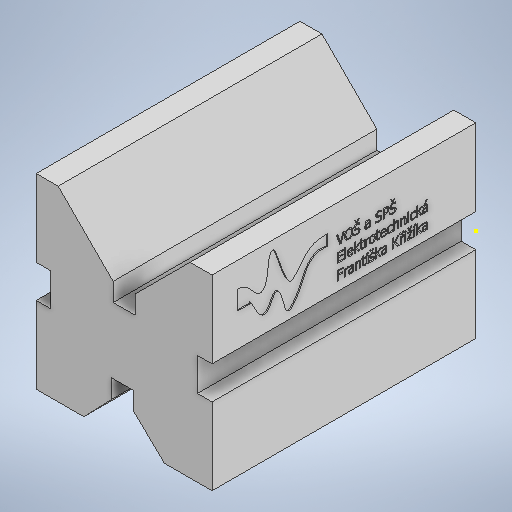
# Autodesk Inventor part: NECO
Saved by Autodesk Inventor 2025 (Build 290162000, 162)
## iProperties
Created: 2025-04-24
Part Number: NECO
Material: Všeobecné
Document SubType Name: Modeling
Designer: jakub
Density: 1 g/cm^3
Appearance: Výchozí
Author: jakub
Autodesk Inventor part; units mm, degrees
(part 1 of 2)
ref_plane "YZ Plane" through (0, 0, 0) normal (1, 0, 0) x (0, 1, 0)
ref_plane "XZ Plane" through (0, 0, 0) normal (0, 1, 0) x (-1, 0, 0)
ref_plane "XY Plane" through (0, 0, 0) normal (0, 0, 1) x (1, 0, 0)
sketch "Sketch1" plane through (0, 0, 0) normal (0, 0, 1) x (1, 0, 0)
  line L0 (0, 4.5) -> (0, 25.5)
  line L1 (0, 4.5) -> (4, 4.5)
  line L2 (4, 4.5) -> (4, 0)
  line L3 (0, 25.5) -> (6, 25.5)
  line L4 (0, 25.5) -> (6, 25.5)
  line L5 (26.7438, 0) -> (4, 0)
  line L6 (6, 25.5) -> (21, 10.5)
  line L7 (48, 4.5) -> (48, 25.5)
  line L8 (48, 4.5) -> (44, 4.5)
  line L9 (44, 4.5) -> (44, 0)
  line L10 (48, 25.5) -> (42, 25.5)
  line L11 (48, 25.5) -> (42, 25.5)
  line L12 (26.7438, 0) -> (44, 0)
  line L13 (42, 25.5) -> (27, 10.5)
  line L14 (24, 5.5) -> (21, 5.5)
  line L15 (21, 5.5) -> (21, 10.5)
  line L16 (24, 5.5) -> (27, 5.5)
  line L17 (27, 5.5) -> (27, 10.5)
  line L18 (4, 0) -> (4, -4.5)
  line L19 (4, -4.5) -> (0, -4.5)
  line L20 (0, 0) -> (0, -25.5)
  line L21 (0, -25.5) -> (48, -25.5)
  line L22 (44, 0) -> (44, -4.5)
  line L23 (44, -4.5) -> (48, -4.5)
  line L24 (48, -4.5) -> (48, -25.5)
  line L25 (0, -25.5) -> (13, -25.5)
  line L26 (13, -25.5) -> (35, -25.5)
  line L27 (20.5688, -12.5) -> (26.5688, -12.5)
  line L28 (13, -25.5) -> (20.5688, -17.6285)
  line L29 (26.5688, -17.3931) -> (35, -25.5)
  line L30 (23.5688, -12.5) -> (26.5688, -12.5)
  line L31 (26.5688, -12.5) -> (26.5688, -17.3931)
  line L32 (23.5688, -12.5) -> (20.5688, -12.5)
  line L33 (20.5688, -12.5) -> (20.5688, -17.6285)
  point P0 (23.7438, 7.7562)
  point P1 (24.2562, 7.7562)
  point P2 (24, -25.5)
  dimension "d0" = 25.5
  dimension "d1" = 4.5
  dimension "d3" = 6
  dimension "d10" = 90
  dimension "d14" = 4.5
  dimension "d15" = 25.5
  dimension "d16" = 48
  dimension "d17" = 13
  dimension "d18" = 22
  dimension "d22" = 90
  dimension "d25" = 6
  dimension "d26" = 13
  constraints: 68 end point, 9 perpendicular, 4 vertical, 3 midpoint, 3 point on line, 1 horizontal, 1 parallel
  measures "d0" distance of L20.start L0.end
  measures "d1" distance of L0.start L20.start
  measures "d3" distance of L3.end L0.end
  measures "d10" angle of L13 L6
  measures "d14" distance of L2.end L18.end
  measures "d15" distance of L20.start L20.end
  measures "d16" distance of L20.end L21.end
  measures "d17" distance of L20.end L25.end
  measures "d18" distance of L25.end L26.end
  measures "d22" angle of L28 L29
  measures "d25" distance of L16.end L14.end
  measures "d26" vertical distance of point (24, -25.5) point (23.569, -12.5)
extrude "Extrusion1" add sketch "Sketch1" along normal blind 72 contours L0 L3 L6 L15 L14 L16 L17 L13 L10 L7 L8 L9 L12 L5 L2 L1 | L5 L12 L22 L23 L24 L21 L29 L31 L27 L33 L28 L20 L19 L18
sketch "Sketch2" plane through (48, 4.5, 0) normal (1, 0, 0) x (0, 0, -1)
  point P0 (0, -4.5)
sketch "Sketch3" plane through (48, 4.5, 0) normal (1, 0, 0) x (0, 0, -1)
  point P0 (0, -4.5)
sketch "Sketch4" plane through (48, 4.5, 0) normal (1, 0, 0) x (0, 0, -1)
  line L0 (-113.7107, -9.1666) -> (-61.0617, -9.1666) construction
  line L1 (-61.0617, -9.1666) -> (-61.0617, -46.8985) construction
  line L2 (-61.0617, -46.8985) -> (-113.7107, -46.8985) construction
  line L3 (-113.7107, -46.8985) -> (-113.7107, -9.1666) construction
  line L4 (-65, 14) -> (-65, 9)
  line L5 (-65, 9) -> (-61.5478, 9)
  line L6 (-40, 12) -> (-42.9346, 12.1178)
  line L7 (-47.0264, 7.7112) -> (-45.9195, 10.8139) construction
  line L8 (-45.9195, 10.8139) -> (-44.0057, 11.8143) construction
  line L9 (-44.0057, 11.8143) -> (-42.9346, 12) construction
  line L10 (-42.9346, 12) -> (-42.9346, 12.1178) construction
  spline S0 degree 4 poles (-47.0264, 7.7112) (-45.9195, 10.8139) (-44.0057, 11.8143) (-42.9346, 12) (-42.9346, 12.1178) knots 1 1 1 1 1 2 2 2 2 2
  spline S1 degree 4 poles (-61.5478, 9) (-61.7679, 11.3374) (-57.3488, -3.3323) (-55.3925, 13.3367) (-52.3539, 5.2468) (-51.4968, -1.6929) (-46.4748, 8.2553) (-46.8368, 8.3647) (-46.4946, 9) knots 0 0 0 0 0 0.346923 0.494972 0.656933 0.800083 1 1 1 1 1
  line L11 (-42.9346, 12) -> (-40.3861, 12.0155)
  line L12 (-40.3861, 12.0155) -> (-40.3861, 15.0416)
  line L13 (-40.3861, 15.0416) -> (-41.6603, 15.0416) construction
  line L14 (-41.6603, 15.0416) -> (-43.7781, 14.867) construction
  line L15 (-43.7781, 14.867) -> (-44.6658, 14.328) construction
  line L16 (-44.6658, 14.328) -> (-46.302, 13.2956) construction
  line L17 (-46.302, 13.2956) -> (-48.14, 11.0974) construction
  line L18 (-48.14, 11.0974) -> (-49.7307, 9) construction
  line L19 (-49.7307, 9) -> (-50.3422, 8.6804) construction
  line L20 (-50.3422, 8.6804) -> (-50.9722, 8.9051) construction
  line L21 (-50.9722, 8.9051) -> (-52.1436, 10.724) construction
  line L22 (-52.1436, 10.724) -> (-53.3658, 14.2638) construction
  line L23 (-53.3658, 14.2638) -> (-54.7945, 18.2323) construction
  line L24 (-54.7945, 18.2323) -> (-55.2231, 18.645) construction
  line L25 (-55.2231, 18.645) -> (-55.6237, 18.645) construction
  line L26 (-55.6237, 18.645) -> (-56.0485, 18.2799) construction
  line L27 (-56.0485, 18.2799) -> (-56.5247, 17.2322) construction
  line L28 (-56.5247, 17.2322) -> (-56.7946, 13.8194) construction
  line L29 (-56.7946, 13.8194) -> (-57.2685, 11.365) construction
  line L30 (-57.2685, 11.365) -> (-58.1756, 10.2319) construction
  line L31 (-58.1756, 10.2319) -> (-58.8495, 10.1151) construction
  line L32 (-58.8495, 10.1151) -> (-59.4762, 10.1151) construction
  line L33 (-59.4762, 10.1151) -> (-60.4296, 11.1367) construction
  line L34 (-60.4296, 11.1367) -> (-61.8566, 12.8776) construction
  line L35 (-61.8566, 12.8776) -> (-63.0012, 13.74) construction
  line L36 (-63.0012, 13.74) -> (-64.3971, 14.238) construction
  line L37 (-64.3971, 14.238) -> (-65, 14.1232) construction
  spline S2 degree 4 poles (-40.3861, 15.0416) (-41.6603, 15.0416) (-43.7781, 14.867) (-44.6658, 14.328) (-46.302, 13.2956) (-48.14, 11.0974) (-49.7307, 9) (-50.3422, 8.6804) (-50.9722, 8.9051) (-52.1436, 10.724) (-53.3658, 14.2638) (-54.7945, 18.2323) (-55.2231, 18.645) (-55.6237, 18.645) (-56.0485, 18.2799) (-56.5247, 17.2322) (-56.7946, 13.8194) (-57.2685, 11.365) (-58.1756, 10.2319) (-58.8495, 10.1151) (-59.4762, 10.1151) (-60.4296, 11.1367) (-61.8566, 12.8776) (-63.0012, 13.74) (-64.3971, 14.238) (-65, 14.1232) knots 1 1 1 1 1 2 3 4 5 6 7 8 9 10 11 12 13 14 15 16 17 18 19 20 21 22 23 23 23 23 23
  line L38 (-65, 14.1232) -> (-65, 14)
  line L39 (-37.9985, 14.2982) -> (-1.01, 14.2982) construction
  line L40 (-1.01, 14.2982) -> (-1.01, 3.2238) construction
  line L41 (-1.01, 3.2238) -> (-37.9985, 3.2238) construction
  line L42 (-37.9985, 3.2238) -> (-37.9985, 14.2982) construction
  line L43 (-35.899, 13.3431) -> (-36.7738, 10.8031)
  line L44 (-36.7738, 10.8031) -> (-37.1381, 10.8031)
  line L45 (-37.1381, 10.8031) -> (-38.0129, 13.3431)
  line L46 (-38.0129, 13.3431) -> (-37.6506, 13.3431)
  line L47 (-37.6506, 13.3431) -> (-36.9467, 11.2333)
  line L48 (-36.9467, 11.2333) -> (-36.2427, 13.3431)
  line L49 (-36.2427, 13.3431) -> (-35.899, 13.3431)
  spline S3 degree 2 poles (-33.8592, 13.0529) (-33.7151, 12.8841) (-33.5545, 12.3901) (-33.5545, 12.0731) knots 0 0 0 1 2 2 2
  spline S4 degree 2 poles (-33.5545, 12.0731) (-33.5545, 11.7644) (-33.711, 11.2642) (-33.8592, 11.0954) knots 0 0 0 1 2 2 2
  spline S5 degree 2 poles (-33.8592, 11.0954) (-34.0156, 10.9184) (-34.4293, 10.7496) (-34.6784, 10.7496) knots 0 0 0 1 2 2 2
  spline S6 degree 2 poles (-34.6784, 10.7496) (-34.9357, 10.7496) (-35.3474, 10.9246) (-35.4976, 11.0954) knots 0 0 0 1 2 2 2
  spline S7 degree 2 poles (-35.4976, 11.0954) (-35.6438, 11.2642) (-35.8002, 11.7602) (-35.8002, 12.0731) knots 0 0 0 1 2 2 2
  spline S8 degree 2 poles (-35.8002, 12.0731) (-35.8002, 12.3922) (-35.6417, 12.8779) (-35.4956, 13.0529) knots 0 0 0 1 2 2 2
  spline S9 degree 2 poles (-35.4956, 13.0529) (-35.3474, 13.2217) (-34.9336, 13.3966) (-34.6784, 13.3966) knots 0 0 0 1 2 2 2
  spline S10 degree 2 poles (-34.6784, 13.3966) (-34.419, 13.3966) (-34.0033, 13.2155) (-33.8592, 13.0529) knots 0 0 0 1 2 2 2
  spline S11 degree 2 poles (-33.9065, 12.0731) (-33.9065, 12.3242) (-34.0156, 12.7133) (-34.1144, 12.8409) knots 0 0 0 1 2 2 2
  spline S12 degree 2 poles (-34.1144, 12.8409) (-34.2153, 12.9726) (-34.4993, 13.1043) (-34.6763, 13.1043) knots 0 0 0 1 2 2 2
  spline S13 degree 2 poles (-34.6763, 13.1043) (-34.8595, 13.1043) (-35.1353, 12.9767) (-35.2403, 12.8409) knots 0 0 0 1 2 2 2
  spline S14 degree 2 poles (-35.2403, 12.8409) (-35.3412, 12.7112) (-35.4482, 12.3201) (-35.4482, 12.0731) knots 0 0 0 1 2 2 2
  spline S15 degree 2 poles (-35.4482, 12.0731) (-35.4482, 11.5729) (-35.0283, 11.0419) (-34.6763, 11.0419) knots 0 0 0 1 2 2 2
  spline S16 degree 2 poles (-34.6763, 11.0419) (-34.3244, 11.0419) (-33.9065, 11.5729) (-33.9065, 12.0731) knots 0 0 0 1 2 2 2
  spline S17 degree 2 poles (-32.476, 10.7578) (-32.7518, 10.7578) (-33.1388, 10.8731) (-33.3096, 10.9554) knots 0 0 0 1 2 2 2
  line L50 (-33.3096, 10.9554) -> (-33.3096, 11.3794)
  line L51 (-33.3096, 11.3794) -> (-33.2849, 11.3794)
  spline S18 degree 2 poles (-33.2849, 11.3794) (-33.1182, 11.223) (-32.6962, 11.0501) (-32.5007, 11.0501) knots 0 0 0 1 2 2 2
  spline S19 degree 2 poles (-32.5007, 11.0501) (-32.2207, 11.0501) (-31.9346, 11.2827) (-31.9346, 11.4741) knots 0 0 0 1 2 2 2
  spline S20 degree 2 poles (-31.9346, 11.4741) (-31.9346, 11.6264) (-32.0849, 11.8158) (-32.2475, 11.8632) knots 0 0 0 1 2 2 2
  spline S21 degree 2 poles (-32.2475, 11.8632) (-32.3648, 11.8961) (-32.5604, 11.9414) (-32.7065, 11.9784) knots 0 0 0 1 2 2 2
  spline S22 degree 2 poles (-32.7065, 11.9784) (-32.8382, 12.0134) (-33.0461, 12.1184) (-33.1264, 12.2028) knots 0 0 0 1 2 2 2
  spline S23 degree 2 poles (-33.1264, 12.2028) (-33.2046, 12.2872) (-33.2911, 12.5136) (-33.2911, 12.6618) knots 0 0 0 1 2 2 2
  spline S24 degree 2 poles (-33.2911, 12.6618) (-33.2911, 12.9705) (-32.8094, 13.3884) (-32.4369, 13.3884) knots 0 0 0 1 2 2 2
  spline S25 degree 2 poles (-32.4369, 13.3884) (-32.2228, 13.3884) (-31.8441, 13.304) (-31.6814, 13.2237) knots 0 0 0 1 2 2 2
  line L52 (-31.6814, 13.2237) -> (-31.6814, 12.8203)
  line L53 (-31.6814, 12.8203) -> (-31.7061, 12.8203)
  spline S26 degree 2 poles (-31.7061, 12.8203) (-31.8276, 12.9314) (-32.2063, 13.0961) (-32.4142, 13.0961) knots 0 0 0 1 2 2 2
  spline S27 degree 2 poles (-32.4142, 13.0961) (-32.6489, 13.0961) (-32.9391, 12.8759) (-32.9391, 12.6968) knots 0 0 0 1 2 2 2
  spline S28 degree 2 poles (-32.9391, 12.6968) (-32.9391, 12.5362) (-32.7682, 12.3448) (-32.6077, 12.3016) knots 0 0 0 1 2 2 2
  spline S29 degree 2 poles (-32.6077, 12.3016) (-32.5007, 12.2728) (-32.1899, 12.1987) (-32.0869, 12.1678) knots 0 0 0 1 2 2 2
  spline S30 degree 2 poles (-32.0869, 12.1678) (-31.8255, 12.0875) (-31.5826, 11.7644) (-31.5826, 11.5276) knots 0 0 0 1 2 2 2
  spline S31 degree 2 poles (-31.5826, 11.5276) (-31.5826, 11.3774) (-31.7041, 11.0892) (-31.8132, 10.9884) knots 0 0 0 1 2 2 2
  spline S32 degree 2 poles (-31.8132, 10.9884) (-31.9346, 10.8772) (-32.2434, 10.7578) (-32.476, 10.7578) knots 0 0 0 1 2 2 2
  line L54 (-31.8585, 14.2982) -> (-32.2475, 13.6519)
  line L55 (-32.2475, 13.6519) -> (-32.6345, 13.6519)
  line L56 (-32.6345, 13.6519) -> (-33.0235, 14.2982)
  line L57 (-33.0235, 14.2982) -> (-32.7518, 14.2982)
  line L58 (-32.7518, 14.2982) -> (-32.4369, 13.8618)
  line L59 (-32.4369, 13.8618) -> (-32.1219, 14.2982)
  line L60 (-32.1219, 14.2982) -> (-31.8585, 14.2982)
  spline S33 degree 2 poles (-29.1106, 11.0048) (-29.1497, 10.976) (-29.2814, 10.8731) (-29.3432, 10.8422) knots 0 0 0 1 2 2 2
  spline S34 degree 2 poles (-29.3432, 10.8422) (-29.4276, 10.7969) (-29.586, 10.7496) (-29.7301, 10.7496) knots 0 0 0 1 2 2 2
  spline S35 degree 2 poles (-29.7301, 10.7496) (-29.8475, 10.7496) (-30.0595, 10.8381) (-30.1397, 10.9184) knots 0 0 0 1 2 2 2
  spline S36 degree 2 poles (-30.1397, 10.9184) (-30.2159, 10.9966) (-30.3085, 11.2271) (-30.3085, 11.3547) knots 0 0 0 1 2 2 2
  spline S37 degree 2 poles (-30.3085, 11.3547) (-30.3085, 11.5523) (-30.1418, 11.8323) (-29.9607, 11.9126) knots 0 0 0 1 2 2 2
  spline S38 degree 2 poles (-29.9607, 11.9126) (-29.8001, 11.9867) (-29.3637, 12.0422) (-29.1106, 12.0566) knots 0 0 0 1 2 2 2
  line L61 (-29.1106, 12.0566) -> (-29.1106, 12.1184)
  spline S39 degree 2 poles (-29.1106, 12.1184) (-29.1106, 12.2295) (-29.1785, 12.3675) (-29.2402, 12.4066) knots 0 0 0 1 2 2 2
  spline S40 degree 2 poles (-29.2402, 12.4066) (-29.302, 12.4457) (-29.479, 12.4704) (-29.5737, 12.4704) knots 0 0 0 1 2 2 2
  spline S41 degree 2 poles (-29.5737, 12.4704) (-29.6848, 12.4704) (-29.9854, 12.4045) (-30.1356, 12.3407) knots 0 0 0 1 2 2 2
  line L62 (-30.1356, 12.3407) -> (-30.1541, 12.3407)
  line L63 (-30.1541, 12.3407) -> (-30.1541, 12.668)
  spline S42 degree 2 poles (-30.1541, 12.668) (-30.0656, 12.6927) (-29.7342, 12.7544) (-29.5716, 12.7544) knots 0 0 0 1 2 2 2
  spline S43 degree 2 poles (-29.5716, 12.7544) (-29.374, 12.7544) (-29.1044, 12.6927) (-28.9974, 12.6124) knots 0 0 0 1 2 2 2
  spline S44 degree 2 poles (-28.9974, 12.6124) (-28.8924, 12.5342) (-28.7895, 12.2851) (-28.7895, 12.106) knots 0 0 0 1 2 2 2
  line L64 (-28.7895, 12.106) -> (-28.7895, 10.8031)
  line L65 (-28.7895, 10.8031) -> (-29.1106, 10.8031)
  line L66 (-29.1106, 10.8031) -> (-29.1106, 11.0048)
  line L67 (-29.1106, 11.2724) -> (-29.1106, 11.8014)
  spline S45 degree 2 poles (-29.1106, 11.8014) (-29.2258, 11.7911) (-29.5737, 11.7561) (-29.6828, 11.7232) knots 0 0 0 1 2 2 2
  spline S46 degree 2 poles (-29.6828, 11.7232) (-29.8104, 11.6841) (-29.9771, 11.5215) (-29.9771, 11.3774) knots 0 0 0 1 2 2 2
  spline S47 degree 2 poles (-29.9771, 11.3774) (-29.9771, 11.2127) (-29.7919, 11.046) (-29.6149, 11.046) knots 0 0 0 1 2 2 2
  spline S48 degree 2 poles (-29.6149, 11.046) (-29.4646, 11.046) (-29.2176, 11.1757) (-29.1106, 11.2724) knots 0 0 0 1 2 2 2
  spline S49 degree 2 poles (-26.515, 10.7578) (-26.7908, 10.7578) (-27.1778, 10.8731) (-27.3486, 10.9554) knots 0 0 0 1 2 2 2
  line L68 (-27.3486, 10.9554) -> (-27.3486, 11.3794)
  line L69 (-27.3486, 11.3794) -> (-27.3239, 11.3794)
  spline S50 degree 2 poles (-27.3239, 11.3794) (-27.1572, 11.223) (-26.7352, 11.0501) (-26.5397, 11.0501) knots 0 0 0 1 2 2 2
  spline S51 degree 2 poles (-26.5397, 11.0501) (-26.2598, 11.0501) (-25.9736, 11.2827) (-25.9736, 11.4741) knots 0 0 0 1 2 2 2
  spline S52 degree 2 poles (-25.9736, 11.4741) (-25.9736, 11.6264) (-26.1239, 11.8158) (-26.2865, 11.8632) knots 0 0 0 1 2 2 2
  spline S53 degree 2 poles (-26.2865, 11.8632) (-26.4038, 11.8961) (-26.5994, 11.9414) (-26.7455, 11.9784) knots 0 0 0 1 2 2 2
  spline S54 degree 2 poles (-26.7455, 11.9784) (-26.8773, 12.0134) (-27.0852, 12.1184) (-27.1654, 12.2028) knots 0 0 0 1 2 2 2
  spline S55 degree 2 poles (-27.1654, 12.2028) (-27.2436, 12.2872) (-27.3301, 12.5136) (-27.3301, 12.6618) knots 0 0 0 1 2 2 2
  spline S56 degree 2 poles (-27.3301, 12.6618) (-27.3301, 12.9705) (-26.8484, 13.3884) (-26.4759, 13.3884) knots 0 0 0 1 2 2 2
  spline S57 degree 2 poles (-26.4759, 13.3884) (-26.2618, 13.3884) (-25.8831, 13.304) (-25.7205, 13.2237) knots 0 0 0 1 2 2 2
  line L70 (-25.7205, 13.2237) -> (-25.7205, 12.8203)
  line L71 (-25.7205, 12.8203) -> (-25.7452, 12.8203)
  spline S58 degree 2 poles (-25.7452, 12.8203) (-25.8666, 12.9314) (-26.2453, 13.0961) (-26.4532, 13.0961) knots 0 0 0 1 2 2 2
  spline S59 degree 2 poles (-26.4532, 13.0961) (-26.6879, 13.0961) (-26.9781, 12.8759) (-26.9781, 12.6968) knots 0 0 0 1 2 2 2
  spline S60 degree 2 poles (-26.9781, 12.6968) (-26.9781, 12.5362) (-26.8073, 12.3448) (-26.6467, 12.3016) knots 0 0 0 1 2 2 2
  spline S61 degree 2 poles (-26.6467, 12.3016) (-26.5397, 12.2728) (-26.2289, 12.1987) (-26.126, 12.1678) knots 0 0 0 1 2 2 2
  spline S62 degree 2 poles (-26.126, 12.1678) (-25.8646, 12.0875) (-25.6217, 11.7644) (-25.6217, 11.5276) knots 0 0 0 1 2 2 2
  spline S63 degree 2 poles (-25.6217, 11.5276) (-25.6217, 11.3774) (-25.7431, 11.0892) (-25.8522, 10.9884) knots 0 0 0 1 2 2 2
  spline S64 degree 2 poles (-25.8522, 10.9884) (-25.9736, 10.8772) (-26.2824, 10.7578) (-26.515, 10.7578) knots 0 0 0 1 2 2 2
  spline S65 degree 2 poles (-23.6724, 12.5774) (-23.6724, 12.4127) (-23.7897, 12.1163) (-23.8947, 12.0134) knots 0 0 0 1 2 2 2
  spline S66 degree 2 poles (-23.8947, 12.0134) (-24.0264, 11.8837) (-24.3825, 11.7499) (-24.6542, 11.7499) knots 0 0 0 1 2 2 2
  line L72 (-24.6542, 11.7499) -> (-24.9404, 11.7499)
  line L73 (-24.9404, 11.7499) -> (-24.9404, 10.8031)
  line L74 (-24.9404, 10.8031) -> (-25.2779, 10.8031)
  line L75 (-25.2779, 10.8031) -> (-25.2779, 13.3431)
  line L76 (-25.2779, 13.3431) -> (-24.6398, 13.3431)
  spline S67 degree 2 poles (-24.6398, 13.3431) (-24.4134, 13.3431) (-24.0964, 13.269) (-23.975, 13.1846) knots 0 0 0 1 2 2 2
  spline S68 degree 2 poles (-23.975, 13.1846) (-23.833, 13.0879) (-23.6724, 12.7894) (-23.6724, 12.5774) knots 0 0 0 1 2 2 2
  spline S69 degree 2 poles (-24.0244, 12.5671) (-24.0244, 12.6988) (-24.115, 12.8923) (-24.2076, 12.9541) knots 0 0 0 1 2 2 2
  spline S70 degree 2 poles (-24.2076, 12.9541) (-24.2879, 13.0076) (-24.5019, 13.0508) (-24.6604, 13.0508) knots 0 0 0 1 2 2 2
  line L77 (-24.6604, 13.0508) -> (-24.9404, 13.0508)
  line L78 (-24.9404, 13.0508) -> (-24.9404, 12.0381)
  line L79 (-24.9404, 12.0381) -> (-24.7098, 12.0381)
  spline S71 degree 2 poles (-24.7098, 12.0381) (-24.504, 12.0381) (-24.2508, 12.104) (-24.1685, 12.1904) knots 0 0 0 1 2 2 2
  spline S72 degree 2 poles (-24.1685, 12.1904) (-24.0923, 12.2666) (-24.0244, 12.4457) (-24.0244, 12.5671) knots 0 0 0 1 2 2 2
  spline S73 degree 2 poles (-22.6432, 10.7578) (-22.9191, 10.7578) (-23.306, 10.8731) (-23.4769, 10.9554) knots 0 0 0 1 2 2 2
  line L80 (-23.4769, 10.9554) -> (-23.4769, 11.3794)
  line L81 (-23.4769, 11.3794) -> (-23.4522, 11.3794)
  spline S74 degree 2 poles (-23.4522, 11.3794) (-23.2854, 11.223) (-22.8635, 11.0501) (-22.6679, 11.0501) knots 0 0 0 1 2 2 2
  spline S75 degree 2 poles (-22.6679, 11.0501) (-22.388, 11.0501) (-22.1019, 11.2827) (-22.1019, 11.4741) knots 0 0 0 1 2 2 2
  spline S76 degree 2 poles (-22.1019, 11.4741) (-22.1019, 11.6264) (-22.2522, 11.8158) (-22.4148, 11.8632) knots 0 0 0 1 2 2 2
  spline S77 degree 2 poles (-22.4148, 11.8632) (-22.5321, 11.8961) (-22.7276, 11.9414) (-22.8738, 11.9784) knots 0 0 0 1 2 2 2
  spline S78 degree 2 poles (-22.8738, 11.9784) (-23.0055, 12.0134) (-23.2134, 12.1184) (-23.2937, 12.2028) knots 0 0 0 1 2 2 2
  spline S79 degree 2 poles (-23.2937, 12.2028) (-23.3719, 12.2872) (-23.4583, 12.5136) (-23.4583, 12.6618) knots 0 0 0 1 2 2 2
  spline S80 degree 2 poles (-23.4583, 12.6618) (-23.4583, 12.9705) (-22.9767, 13.3884) (-22.6041, 13.3884) knots 0 0 0 1 2 2 2
  spline S81 degree 2 poles (-22.6041, 13.3884) (-22.3901, 13.3884) (-22.0113, 13.304) (-21.8487, 13.2237) knots 0 0 0 1 2 2 2
  line L82 (-21.8487, 13.2237) -> (-21.8487, 12.8203)
  line L83 (-21.8487, 12.8203) -> (-21.8734, 12.8203)
  spline S82 degree 2 poles (-21.8734, 12.8203) (-21.9949, 12.9314) (-22.3736, 13.0961) (-22.5815, 13.0961) knots 0 0 0 1 2 2 2
  spline S83 degree 2 poles (-22.5815, 13.0961) (-22.8161, 13.0961) (-23.1064, 12.8759) (-23.1064, 12.6968) knots 0 0 0 1 2 2 2
  spline S84 degree 2 poles (-23.1064, 12.6968) (-23.1064, 12.5362) (-22.9355, 12.3448) (-22.775, 12.3016) knots 0 0 0 1 2 2 2
  spline S85 degree 2 poles (-22.775, 12.3016) (-22.6679, 12.2728) (-22.3571, 12.1987) (-22.2542, 12.1678) knots 0 0 0 1 2 2 2
  spline S86 degree 2 poles (-22.2542, 12.1678) (-21.9928, 12.0875) (-21.7499, 11.7644) (-21.7499, 11.5276) knots 0 0 0 1 2 2 2
  spline S87 degree 2 poles (-21.7499, 11.5276) (-21.7499, 11.3774) (-21.8714, 11.0892) (-21.9805, 10.9884) knots 0 0 0 1 2 2 2
  spline S88 degree 2 poles (-21.9805, 10.9884) (-22.1019, 10.8772) (-22.4106, 10.7578) (-22.6432, 10.7578) knots 0 0 0 1 2 2 2
  line L84 (-22.0257, 14.2982) -> (-22.4148, 13.6519)
  line L85 (-22.4148, 13.6519) -> (-22.8017, 13.6519)
  line L86 (-22.8017, 13.6519) -> (-23.1908, 14.2982)
  line L87 (-23.1908, 14.2982) -> (-22.9191, 14.2982)
  line L88 (-22.9191, 14.2982) -> (-22.6041, 13.8618)
  line L89 (-22.6041, 13.8618) -> (-22.2892, 14.2982)
  line L90 (-22.2892, 14.2982) -> (-22.0257, 14.2982)
  line L91 (-37.7412, 6.6211) -> (-37.7412, 9.1611)
  line L92 (-37.7412, 9.1611) -> (-36.1522, 9.1611)
  line L93 (-36.1522, 9.1611) -> (-36.1522, 8.8605)
  line L94 (-36.1522, 8.8605) -> (-37.4036, 8.8605)
  line L95 (-37.4036, 8.8605) -> (-37.4036, 8.1648)
  line L96 (-37.4036, 8.1648) -> (-36.2366, 8.1648)
  line L97 (-36.2366, 8.1648) -> (-36.2366, 7.8643)
  line L98 (-36.2366, 7.8643) -> (-37.4036, 7.8643)
  line L99 (-37.4036, 7.8643) -> (-37.4036, 6.9216)
  line L100 (-37.4036, 6.9216) -> (-36.1522, 6.9216)
  line L101 (-36.1522, 6.9216) -> (-36.1522, 6.6211)
  line L102 (-36.1522, 6.6211) -> (-37.7412, 6.6211)
  line L103 (-35.4791, 6.6211) -> (-35.8002, 6.6211)
  line L104 (-35.8002, 6.6211) -> (-35.8002, 9.2743)
  line L105 (-35.8002, 9.2743) -> (-35.4791, 9.2743)
  line L106 (-35.4791, 9.2743) -> (-35.4791, 6.6211)
  spline S89 degree 2 poles (-34.1803, 6.5778) (-34.6372, 6.5778) (-35.1395, 7.0904) (-35.1395, 7.5638) knots 0 0 0 1 2 2 2
  spline S90 degree 2 poles (-35.1395, 7.5638) (-35.1395, 8.029) (-34.6516, 8.5806) (-34.2585, 8.5806) knots 0 0 0 1 2 2 2
  spline S91 degree 2 poles (-34.2585, 8.5806) (-34.0815, 8.5806) (-33.8077, 8.4777) (-33.7069, 8.3686) knots 0 0 0 1 2 2 2
  spline S92 degree 2 poles (-33.7069, 8.3686) (-33.6039, 8.2595) (-33.4948, 7.9446) (-33.4948, 7.7161) knots 0 0 0 1 2 2 2
  line L107 (-33.4948, 7.7161) -> (-33.4948, 7.5411)
  line L108 (-33.4948, 7.5411) -> (-34.8142, 7.5411)
  spline S93 degree 2 poles (-34.8142, 7.5411) (-34.8142, 7.2098) (-34.4808, 6.8578) (-34.1844, 6.8578) knots 0 0 0 1 2 2 2
  spline S94 degree 2 poles (-34.1844, 6.8578) (-34.0794, 6.8578) (-33.8756, 6.9051) (-33.7933, 6.9422) knots 0 0 0 1 2 2 2
  spline S95 degree 2 poles (-33.7933, 6.9422) (-33.7069, 6.9833) (-33.5875, 7.0554) (-33.5484, 7.0883) knots 0 0 0 1 2 2 2
  line L109 (-33.5484, 7.0883) -> (-33.5298, 7.0883)
  line L110 (-33.5298, 7.0883) -> (-33.5298, 6.7384)
  spline S96 degree 2 poles (-33.5298, 6.7384) (-33.5854, 6.7158) (-33.7542, 6.6499) (-33.8201, 6.6314) knots 0 0 0 1 2 2 2
  spline S97 degree 2 poles (-33.8201, 6.6314) (-33.9127, 6.6046) (-34.065, 6.5778) (-34.1803, 6.5778) knots 0 0 0 1 2 2 2
  spline S98 degree 2 poles (-33.8077, 7.7861) (-33.8118, 7.9158) (-33.8653, 8.1051) (-33.9168, 8.1689) knots 0 0 0 1 2 2 2
  spline S99 degree 2 poles (-33.9168, 8.1689) (-33.9724, 8.241) (-34.1473, 8.3171) (-34.277, 8.3171) knots 0 0 0 1 2 2 2
  spline S100 degree 2 poles (-34.277, 8.3171) (-34.4046, 8.3171) (-34.5837, 8.241) (-34.6578, 8.1669) knots 0 0 0 1 2 2 2
  spline S101 degree 2 poles (-34.6578, 8.1669) (-34.7299, 8.0907) (-34.804, 7.9075) (-34.8142, 7.7861) knots 0 0 0 1 2 2 2
  line L111 (-34.8142, 7.7861) -> (-33.8077, 7.7861)
  line L112 (-31.5909, 6.6211) -> (-32.0128, 6.6211)
  line L113 (-32.0128, 6.6211) -> (-32.7209, 7.5411)
  line L114 (-32.7209, 7.5411) -> (-32.8485, 7.4176)
  line L115 (-32.8485, 7.4176) -> (-32.8485, 6.6211)
  line L116 (-32.8485, 6.6211) -> (-33.1696, 6.6211)
  line L117 (-33.1696, 6.6211) -> (-33.1696, 9.2743)
  line L118 (-33.1696, 9.2743) -> (-32.8485, 9.2743)
  line L119 (-32.8485, 9.2743) -> (-32.8485, 7.7223)
  line L120 (-32.8485, 7.7223) -> (-32.0952, 8.5271)
  line L121 (-32.0952, 8.5271) -> (-31.6959, 8.5271)
  line L122 (-31.6959, 8.5271) -> (-32.478, 7.7305)
  line L123 (-32.478, 7.7305) -> (-31.5909, 6.6211)
  spline S102 degree 2 poles (-30.854, 6.584) (-31.1154, 6.584) (-31.4097, 6.8825) (-31.4097, 7.2056) knots 0 0 0 1 2 2 2
  line L124 (-31.4097, 7.2056) -> (-31.4097, 8.2616)
  line L125 (-31.4097, 8.2616) -> (-31.6259, 8.2616)
  line L126 (-31.6259, 8.2616) -> (-31.6259, 8.5271)
  line L127 (-31.6259, 8.5271) -> (-31.4097, 8.5271)
  line L128 (-31.4097, 8.5271) -> (-31.4097, 9.0746)
  line L129 (-31.4097, 9.0746) -> (-31.0886, 9.0746)
  line L130 (-31.0886, 9.0746) -> (-31.0886, 8.5271)
  line L131 (-31.0886, 8.5271) -> (-30.4979, 8.5271)
  line L132 (-30.4979, 8.5271) -> (-30.4979, 8.2616)
  line L133 (-30.4979, 8.2616) -> (-31.0886, 8.2616)
  line L134 (-31.0886, 8.2616) -> (-31.0886, 7.3538)
  spline S103 degree 2 poles (-31.0886, 7.3538) (-31.0886, 7.2098) (-31.0783, 7.0513) (-31.0434, 6.9833) knots 0 0 0 1 2 2 2
  spline S104 degree 2 poles (-31.0434, 6.9833) (-31.0145, 6.9236) (-30.8849, 6.864) (-30.7737, 6.864) knots 0 0 0 1 2 2 2
  spline S105 degree 2 poles (-30.7737, 6.864) (-30.6955, 6.864) (-30.5494, 6.9113) (-30.5164, 6.9257) knots 0 0 0 1 2 2 2
  line L135 (-30.5164, 6.9257) -> (-30.4979, 6.9257)
  line L136 (-30.4979, 6.9257) -> (-30.4979, 6.6375)
  spline S106 degree 2 poles (-30.4979, 6.6375) (-30.5885, 6.6128) (-30.7737, 6.584) (-30.854, 6.584) knots 0 0 0 1 2 2 2
  line L137 (-29.2505, 8.1834) -> (-29.267, 8.1834)
  spline S107 degree 2 poles (-29.267, 8.1834) (-29.3041, 8.1936) (-29.3843, 8.1978) (-29.4399, 8.1978) knots 0 0 0 1 2 2 2
  spline S108 degree 2 poles (-29.4399, 8.1978) (-29.5696, 8.1978) (-29.8248, 8.0846) (-29.9401, 7.9734) knots 0 0 0 1 2 2 2
  line L138 (-29.9401, 7.9734) -> (-29.9401, 6.6211)
  line L139 (-29.9401, 6.6211) -> (-30.2612, 6.6211)
  line L140 (-30.2612, 6.6211) -> (-30.2612, 8.5271)
  line L141 (-30.2612, 8.5271) -> (-29.9401, 8.5271)
  line L142 (-29.9401, 8.5271) -> (-29.9401, 8.243)
  spline S109 degree 2 poles (-29.9401, 8.243) (-29.7651, 8.3995) (-29.5037, 8.5271) (-29.3802, 8.5271) knots 0 0 0 1 2 2 2
  spline S110 degree 2 poles (-29.3802, 8.5271) (-29.3308, 8.5271) (-29.2814, 8.523) (-29.2505, 8.5168) knots 0 0 0 1 2 2 2
  line L143 (-29.2505, 8.5168) -> (-29.2505, 8.1834)
  spline S111 degree 2 poles (-27.4351, 7.5741) (-27.4351, 7.0924) (-27.8982, 6.5675) (-28.2852, 6.5675) knots 0 0 0 1 2 2 2
  spline S112 degree 2 poles (-28.2852, 6.5675) (-28.6824, 6.5675) (-29.1373, 7.1089) (-29.1373, 7.5741) knots 0 0 0 1 2 2 2
  spline S113 degree 2 poles (-29.1373, 7.5741) (-29.1373, 8.0516) (-28.668, 8.5806) (-28.2852, 8.5806) knots 0 0 0 1 2 2 2
  spline S114 degree 2 poles (-28.2852, 8.5806) (-27.8982, 8.5806) (-27.4351, 8.0537) (-27.4351, 7.5741) knots 0 0 0 1 2 2 2
  spline S115 degree 2 poles (-27.7665, 7.5741) (-27.7665, 7.9446) (-28.0361, 8.3048) (-28.2852, 8.3048) knots 0 0 0 1 2 2 2
  spline S116 degree 2 poles (-28.2852, 8.3048) (-28.5342, 8.3048) (-28.8059, 7.9446) (-28.8059, 7.5741) knots 0 0 0 1 2 2 2
  spline S117 degree 2 poles (-28.8059, 7.5741) (-28.8059, 7.2139) (-28.5342, 6.8434) (-28.2852, 6.8434) knots 0 0 0 1 2 2 2
  spline S118 degree 2 poles (-28.2852, 6.8434) (-28.0382, 6.8434) (-27.7665, 7.2077) (-27.7665, 7.5741) knots 0 0 0 1 2 2 2
  spline S119 degree 2 poles (-26.5294, 6.584) (-26.7908, 6.584) (-27.0852, 6.8825) (-27.0852, 7.2056) knots 0 0 0 1 2 2 2
  line L144 (-27.0852, 7.2056) -> (-27.0852, 8.2616)
  line L145 (-27.0852, 8.2616) -> (-27.3013, 8.2616)
  line L146 (-27.3013, 8.2616) -> (-27.3013, 8.5271)
  line L147 (-27.3013, 8.5271) -> (-27.0852, 8.5271)
  line L148 (-27.0852, 8.5271) -> (-27.0852, 9.0746)
  line L149 (-27.0852, 9.0746) -> (-26.7641, 9.0746)
  line L150 (-26.7641, 9.0746) -> (-26.7641, 8.5271)
  line L151 (-26.7641, 8.5271) -> (-26.1733, 8.5271)
  line L152 (-26.1733, 8.5271) -> (-26.1733, 8.2616)
  line L153 (-26.1733, 8.2616) -> (-26.7641, 8.2616)
  line L154 (-26.7641, 8.2616) -> (-26.7641, 7.3538)
  spline S120 degree 2 poles (-26.7641, 7.3538) (-26.7641, 7.2098) (-26.7538, 7.0513) (-26.7188, 6.9833) knots 0 0 0 1 2 2 2
  spline S121 degree 2 poles (-26.7188, 6.9833) (-26.69, 6.9236) (-26.5603, 6.864) (-26.4491, 6.864) knots 0 0 0 1 2 2 2
  spline S122 degree 2 poles (-26.4491, 6.864) (-26.3709, 6.864) (-26.2248, 6.9113) (-26.1918, 6.9257) knots 0 0 0 1 2 2 2
  line L155 (-26.1918, 6.9257) -> (-26.1733, 6.9257)
  line L156 (-26.1733, 6.9257) -> (-26.1733, 6.6375)
  spline S123 degree 2 poles (-26.1733, 6.6375) (-26.2639, 6.6128) (-26.4491, 6.584) (-26.5294, 6.584) knots 0 0 0 1 2 2 2
  spline S124 degree 2 poles (-25.1091, 6.5778) (-25.5661, 6.5778) (-26.0683, 7.0904) (-26.0683, 7.5638) knots 0 0 0 1 2 2 2
  spline S125 degree 2 poles (-26.0683, 7.5638) (-26.0683, 8.029) (-25.5805, 8.5806) (-25.1874, 8.5806) knots 0 0 0 1 2 2 2
  spline S126 degree 2 poles (-25.1874, 8.5806) (-25.0103, 8.5806) (-24.7366, 8.4777) (-24.6357, 8.3686) knots 0 0 0 1 2 2 2
  spline S127 degree 2 poles (-24.6357, 8.3686) (-24.5328, 8.2595) (-24.4237, 7.9446) (-24.4237, 7.7161) knots 0 0 0 1 2 2 2
  line L157 (-24.4237, 7.7161) -> (-24.4237, 7.5411)
  line L158 (-24.4237, 7.5411) -> (-25.7431, 7.5411)
  spline S128 degree 2 poles (-25.7431, 7.5411) (-25.7431, 7.2098) (-25.4097, 6.8578) (-25.1133, 6.8578) knots 0 0 0 1 2 2 2
  spline S129 degree 2 poles (-25.1133, 6.8578) (-25.0083, 6.8578) (-24.8045, 6.9051) (-24.7222, 6.9422) knots 0 0 0 1 2 2 2
  spline S130 degree 2 poles (-24.7222, 6.9422) (-24.6357, 6.9833) (-24.5163, 7.0554) (-24.4772, 7.0883) knots 0 0 0 1 2 2 2
  line L159 (-24.4772, 7.0883) -> (-24.4587, 7.0883)
  line L160 (-24.4587, 7.0883) -> (-24.4587, 6.7384)
  spline S131 degree 2 poles (-24.4587, 6.7384) (-24.5143, 6.7158) (-24.6831, 6.6499) (-24.7489, 6.6314) knots 0 0 0 1 2 2 2
  spline S132 degree 2 poles (-24.7489, 6.6314) (-24.8416, 6.6046) (-24.9939, 6.5778) (-25.1091, 6.5778) knots 0 0 0 1 2 2 2
  spline S133 degree 2 poles (-24.7366, 7.7861) (-24.7407, 7.9158) (-24.7942, 8.1051) (-24.8457, 8.1689) knots 0 0 0 1 2 2 2
  spline S134 degree 2 poles (-24.8457, 8.1689) (-24.9012, 8.241) (-25.0762, 8.3171) (-25.2059, 8.3171) knots 0 0 0 1 2 2 2
  spline S135 degree 2 poles (-25.2059, 8.3171) (-25.3335, 8.3171) (-25.5126, 8.241) (-25.5867, 8.1669) knots 0 0 0 1 2 2 2
  spline S136 degree 2 poles (-25.5867, 8.1669) (-25.6587, 8.0907) (-25.7328, 7.9075) (-25.7431, 7.7861) knots 0 0 0 1 2 2 2
  line L161 (-25.7431, 7.7861) -> (-24.7366, 7.7861)
  spline S137 degree 2 poles (-23.341, 6.5778) (-23.5386, 6.5778) (-23.8659, 6.6993) (-23.9832, 6.8228) knots 0 0 0 1 2 2 2
  spline S138 degree 2 poles (-23.9832, 6.8228) (-24.1006, 6.9442) (-24.2302, 7.3188) (-24.2302, 7.57) knots 0 0 0 1 2 2 2
  spline S139 degree 2 poles (-24.2302, 7.57) (-24.2302, 7.8211) (-24.0964, 8.1875) (-23.9832, 8.311) knots 0 0 0 1 2 2 2
  spline S140 degree 2 poles (-23.9832, 8.311) (-23.87, 8.4365) (-23.5345, 8.5703) (-23.341, 8.5703) knots 0 0 0 1 2 2 2
  spline S141 degree 2 poles (-23.341, 8.5703) (-23.1846, 8.5703) (-22.8923, 8.4818) (-22.7791, 8.4242) knots 0 0 0 1 2 2 2
  line L162 (-22.7791, 8.4242) -> (-22.7791, 8.064)
  line L163 (-22.7791, 8.064) -> (-22.7976, 8.064)
  spline S142 degree 2 poles (-22.7976, 8.064) (-22.8326, 8.0928) (-22.9396, 8.1669) (-23.0158, 8.206) knots 0 0 0 1 2 2 2
  spline S143 degree 2 poles (-23.0158, 8.206) (-23.0837, 8.2389) (-23.2649, 8.2904) (-23.3472, 8.2904) knots 0 0 0 1 2 2 2
  spline S144 degree 2 poles (-23.3472, 8.2904) (-23.5963, 8.2904) (-23.8988, 7.9137) (-23.8988, 7.57) knots 0 0 0 1 2 2 2
  spline S145 degree 2 poles (-23.8988, 7.57) (-23.8988, 7.2345) (-23.6065, 6.8578) (-23.3472, 6.8578) knots 0 0 0 1 2 2 2
  spline S146 degree 2 poles (-23.3472, 6.8578) (-23.1908, 6.8578) (-22.9067, 6.9875) (-22.7976, 7.0883) knots 0 0 0 1 2 2 2
  line L164 (-22.7976, 7.0883) -> (-22.7791, 7.0883)
  line L165 (-22.7791, 7.0883) -> (-22.7791, 6.7281)
  spline S147 degree 2 poles (-22.7791, 6.7281) (-22.8264, 6.7055) (-22.9705, 6.6416) (-23.0282, 6.6272) knots 0 0 0 1 2 2 2
  spline S148 degree 2 poles (-23.0282, 6.6272) (-23.1105, 6.6025) (-23.2402, 6.5778) (-23.341, 6.5778) knots 0 0 0 1 2 2 2
  line L166 (-20.9904, 6.6211) -> (-21.3115, 6.6211)
  line L167 (-21.3115, 6.6211) -> (-21.3115, 7.7079)
  spline S149 degree 2 poles (-21.3115, 7.7079) (-21.3115, 7.8396) (-21.3362, 8.066) (-21.3732, 8.134) knots 0 0 0 1 2 2 2
  spline S150 degree 2 poles (-21.3732, 8.134) (-21.4123, 8.206) (-21.5523, 8.276) (-21.6717, 8.276) knots 0 0 0 1 2 2 2
  spline S151 degree 2 poles (-21.6717, 8.276) (-21.7911, 8.276) (-22.0443, 8.1484) (-22.1657, 8.0454) knots 0 0 0 1 2 2 2
  line L168 (-22.1657, 8.0454) -> (-22.1657, 6.6211)
  line L169 (-22.1657, 6.6211) -> (-22.4868, 6.6211)
  line L170 (-22.4868, 6.6211) -> (-22.4868, 9.2743)
  line L171 (-22.4868, 9.2743) -> (-22.1657, 9.2743)
  line L172 (-22.1657, 9.2743) -> (-22.1657, 8.3151)
  spline S152 degree 2 poles (-22.1657, 8.3151) (-22.0216, 8.4448) (-21.7437, 8.5806) (-21.5873, 8.5806) knots 0 0 0 1 2 2 2
  spline S153 degree 2 poles (-21.5873, 8.5806) (-21.3074, 8.5806) (-20.9904, 8.2101) (-20.9904, 7.8581) knots 0 0 0 1 2 2 2
  line L173 (-20.9904, 7.8581) -> (-20.9904, 6.6211)
  line L174 (-19.0432, 6.6211) -> (-19.3643, 6.6211)
  line L175 (-19.3643, 6.6211) -> (-19.3643, 7.7079)
  spline S154 degree 2 poles (-19.3643, 7.7079) (-19.3643, 7.8396) (-19.389, 8.066) (-19.426, 8.134) knots 0 0 0 1 2 2 2
  spline S155 degree 2 poles (-19.426, 8.134) (-19.4652, 8.206) (-19.6051, 8.276) (-19.7245, 8.276) knots 0 0 0 1 2 2 2
  spline S156 degree 2 poles (-19.7245, 8.276) (-19.8439, 8.276) (-20.0971, 8.1484) (-20.2185, 8.0454) knots 0 0 0 1 2 2 2
  line L176 (-20.2185, 8.0454) -> (-20.2185, 6.6211)
  line L177 (-20.2185, 6.6211) -> (-20.5396, 6.6211)
  line L178 (-20.5396, 6.6211) -> (-20.5396, 8.5271)
  line L179 (-20.5396, 8.5271) -> (-20.2185, 8.5271)
  line L180 (-20.2185, 8.5271) -> (-20.2185, 8.3151)
  spline S157 degree 2 poles (-20.2185, 8.3151) (-20.0744, 8.4448) (-19.7965, 8.5806) (-19.6401, 8.5806) knots 0 0 0 1 2 2 2
  spline S158 degree 2 poles (-19.6401, 8.5806) (-19.3602, 8.5806) (-19.0432, 8.2101) (-19.0432, 7.8581) knots 0 0 0 1 2 2 2
  line L181 (-19.0432, 7.8581) -> (-19.0432, 6.6211)
  line L182 (-18.2651, 6.6211) -> (-18.5862, 6.6211)
  line L183 (-18.5862, 6.6211) -> (-18.5862, 8.5271)
  line L184 (-18.5862, 8.5271) -> (-18.2651, 8.5271)
  line L185 (-18.2651, 8.5271) -> (-18.2651, 6.6211)
  line L186 (-18.2425, 8.8441) -> (-18.6068, 8.8441)
  line L187 (-18.6068, 8.8441) -> (-18.6068, 9.1775)
  line L188 (-18.6068, 9.1775) -> (-18.2425, 9.1775)
  line L189 (-18.2425, 9.1775) -> (-18.2425, 8.8441)
  spline S159 degree 2 poles (-17.0363, 6.5778) (-17.2339, 6.5778) (-17.5612, 6.6993) (-17.6785, 6.8228) knots 0 0 0 1 2 2 2
  spline S160 degree 2 poles (-17.6785, 6.8228) (-17.7958, 6.9442) (-17.9255, 7.3188) (-17.9255, 7.57) knots 0 0 0 1 2 2 2
  spline S161 degree 2 poles (-17.9255, 7.57) (-17.9255, 7.8211) (-17.7917, 8.1875) (-17.6785, 8.311) knots 0 0 0 1 2 2 2
  spline S162 degree 2 poles (-17.6785, 8.311) (-17.5653, 8.4365) (-17.2298, 8.5703) (-17.0363, 8.5703) knots 0 0 0 1 2 2 2
  spline S163 degree 2 poles (-17.0363, 8.5703) (-16.8799, 8.5703) (-16.5876, 8.4818) (-16.4744, 8.4242) knots 0 0 0 1 2 2 2
  line L190 (-16.4744, 8.4242) -> (-16.4744, 8.064)
  line L191 (-16.4744, 8.064) -> (-16.4929, 8.064)
  spline S164 degree 2 poles (-16.4929, 8.064) (-16.5279, 8.0928) (-16.6349, 8.1669) (-16.7111, 8.206) knots 0 0 0 1 2 2 2
  spline S165 degree 2 poles (-16.7111, 8.206) (-16.779, 8.2389) (-16.9601, 8.2904) (-17.0425, 8.2904) knots 0 0 0 1 2 2 2
  spline S166 degree 2 poles (-17.0425, 8.2904) (-17.2915, 8.2904) (-17.5941, 7.9137) (-17.5941, 7.57) knots 0 0 0 1 2 2 2
  spline S167 degree 2 poles (-17.5941, 7.57) (-17.5941, 7.2345) (-17.3018, 6.8578) (-17.0425, 6.8578) knots 0 0 0 1 2 2 2
  spline S168 degree 2 poles (-17.0425, 6.8578) (-16.886, 6.8578) (-16.602, 6.9875) (-16.4929, 7.0883) knots 0 0 0 1 2 2 2
  line L192 (-16.4929, 7.0883) -> (-16.4744, 7.0883)
  line L193 (-16.4744, 7.0883) -> (-16.4744, 6.7281)
  spline S169 degree 2 poles (-16.4744, 6.7281) (-16.5217, 6.7055) (-16.6658, 6.6416) (-16.7234, 6.6272) knots 0 0 0 1 2 2 2
  spline S170 degree 2 poles (-16.7234, 6.6272) (-16.8058, 6.6025) (-16.9354, 6.5778) (-17.0363, 6.5778) knots 0 0 0 1 2 2 2
  line L194 (-14.6033, 6.6211) -> (-15.0253, 6.6211)
  line L195 (-15.0253, 6.6211) -> (-15.7334, 7.5411)
  line L196 (-15.7334, 7.5411) -> (-15.861, 7.4176)
  line L197 (-15.861, 7.4176) -> (-15.861, 6.6211)
  line L198 (-15.861, 6.6211) -> (-16.1821, 6.6211)
  line L199 (-16.1821, 6.6211) -> (-16.1821, 9.2743)
  line L200 (-16.1821, 9.2743) -> (-15.861, 9.2743)
  line L201 (-15.861, 9.2743) -> (-15.861, 7.7223)
  line L202 (-15.861, 7.7223) -> (-15.1076, 8.5271)
  line L203 (-15.1076, 8.5271) -> (-14.7083, 8.5271)
  line L204 (-14.7083, 8.5271) -> (-15.4905, 7.7305)
  line L205 (-15.4905, 7.7305) -> (-14.6033, 6.6211)
  spline S171 degree 2 poles (-13.3807, 6.8228) (-13.4198, 6.794) (-13.5515, 6.6911) (-13.6133, 6.6602) knots 0 0 0 1 2 2 2
  spline S172 degree 2 poles (-13.6133, 6.6602) (-13.6977, 6.6149) (-13.8562, 6.5675) (-14.0002, 6.5675) knots 0 0 0 1 2 2 2
  spline S173 degree 2 poles (-14.0002, 6.5675) (-14.1176, 6.5675) (-14.3296, 6.6561) (-14.4099, 6.7363) knots 0 0 0 1 2 2 2
  spline S174 degree 2 poles (-14.4099, 6.7363) (-14.486, 6.8146) (-14.5786, 7.0451) (-14.5786, 7.1727) knots 0 0 0 1 2 2 2
  spline S175 degree 2 poles (-14.5786, 7.1727) (-14.5786, 7.3703) (-14.4119, 7.6502) (-14.2308, 7.7305) knots 0 0 0 1 2 2 2
  spline S176 degree 2 poles (-14.2308, 7.7305) (-14.0702, 7.8046) (-13.6339, 7.8602) (-13.3807, 7.8746) knots 0 0 0 1 2 2 2
  line L206 (-13.3807, 7.8746) -> (-13.3807, 7.9363)
  spline S177 degree 2 poles (-13.3807, 7.9363) (-13.3807, 8.0475) (-13.4486, 8.1854) (-13.5104, 8.2245) knots 0 0 0 1 2 2 2
  spline S178 degree 2 poles (-13.5104, 8.2245) (-13.5721, 8.2636) (-13.7491, 8.2883) (-13.8438, 8.2883) knots 0 0 0 1 2 2 2
  spline S179 degree 2 poles (-13.8438, 8.2883) (-13.955, 8.2883) (-14.2555, 8.2225) (-14.4057, 8.1587) knots 0 0 0 1 2 2 2
  line L207 (-14.4057, 8.1587) -> (-14.4243, 8.1587)
  line L208 (-14.4243, 8.1587) -> (-14.4243, 8.4859)
  spline S180 degree 2 poles (-14.4243, 8.4859) (-14.3358, 8.5106) (-14.0044, 8.5724) (-13.8417, 8.5724) knots 0 0 0 1 2 2 2
  spline S181 degree 2 poles (-13.8417, 8.5724) (-13.6441, 8.5724) (-13.3745, 8.5106) (-13.2675, 8.4304) knots 0 0 0 1 2 2 2
  spline S182 degree 2 poles (-13.2675, 8.4304) (-13.1625, 8.3521) (-13.0596, 8.1031) (-13.0596, 7.924) knots 0 0 0 1 2 2 2
  line L209 (-13.0596, 7.924) -> (-13.0596, 6.6211)
  line L210 (-13.0596, 6.6211) -> (-13.3807, 6.6211)
  line L211 (-13.3807, 6.6211) -> (-13.3807, 6.8228)
  line L212 (-13.3807, 7.0904) -> (-13.3807, 7.6194)
  spline S183 degree 2 poles (-13.3807, 7.6194) (-13.4959, 7.6091) (-13.8438, 7.5741) (-13.9529, 7.5411) knots 0 0 0 1 2 2 2
  spline S184 degree 2 poles (-13.9529, 7.5411) (-14.0805, 7.502) (-14.2472, 7.3394) (-14.2472, 7.1953) knots 0 0 0 1 2 2 2
  spline S185 degree 2 poles (-14.2472, 7.1953) (-14.2472, 7.0307) (-14.062, 6.864) (-13.885, 6.864) knots 0 0 0 1 2 2 2
  spline S186 degree 2 poles (-13.885, 6.864) (-13.7347, 6.864) (-13.4877, 6.9936) (-13.3807, 7.0904) knots 0 0 0 1 2 2 2
  line L213 (-13.2489, 9.4801) -> (-13.7141, 8.842)
  line L214 (-13.7141, 8.842) -> (-13.9694, 8.842)
  line L215 (-13.9694, 8.842) -> (-13.6647, 9.4801)
  line L216 (-13.6647, 9.4801) -> (-13.2489, 9.4801)
  line L217 (-36.2222, 4.6785) -> (-37.4036, 4.6785)
  line L218 (-37.4036, 4.6785) -> (-37.4036, 3.9622)
  line L219 (-37.4036, 3.9622) -> (-36.2716, 3.9622)
  line L220 (-36.2716, 3.9622) -> (-36.2716, 3.6617)
  line L221 (-36.2716, 3.6617) -> (-37.4036, 3.6617)
  line L222 (-37.4036, 3.6617) -> (-37.4036, 2.439)
  line L223 (-37.4036, 2.439) -> (-37.7412, 2.439)
  line L224 (-37.7412, 2.439) -> (-37.7412, 4.979)
  line L225 (-37.7412, 4.979) -> (-36.2222, 4.979)
  line L226 (-36.2222, 4.979) -> (-36.2222, 4.6785)
  line L227 (-34.9336, 4.0013) -> (-34.9501, 4.0013)
  spline S187 degree 2 poles (-34.9501, 4.0013) (-34.9871, 4.0116) (-35.0674, 4.0157) (-35.123, 4.0157) knots 0 0 0 1 2 2 2
  spline S188 degree 2 poles (-35.123, 4.0157) (-35.2527, 4.0157) (-35.5079, 3.9025) (-35.6232, 3.7914) knots 0 0 0 1 2 2 2
  line L228 (-35.6232, 3.7914) -> (-35.6232, 2.439)
  line L229 (-35.6232, 2.439) -> (-35.9443, 2.439)
  line L230 (-35.9443, 2.439) -> (-35.9443, 4.3451)
  line L231 (-35.9443, 4.3451) -> (-35.6232, 4.3451)
  line L232 (-35.6232, 4.3451) -> (-35.6232, 4.061)
  spline S189 degree 2 poles (-35.6232, 4.061) (-35.4482, 4.2174) (-35.1868, 4.3451) (-35.0633, 4.3451) knots 0 0 0 1 2 2 2
  spline S190 degree 2 poles (-35.0633, 4.3451) (-35.0139, 4.3451) (-34.9645, 4.3409) (-34.9336, 4.3348) knots 0 0 0 1 2 2 2
  line L233 (-34.9336, 4.3348) -> (-34.9336, 4.0013)
  spline S191 degree 2 poles (-33.6225, 2.6407) (-33.6616, 2.6119) (-33.7933, 2.509) (-33.8551, 2.4781) knots 0 0 0 1 2 2 2
  spline S192 degree 2 poles (-33.8551, 2.4781) (-33.9394, 2.4328) (-34.0979, 2.3855) (-34.242, 2.3855) knots 0 0 0 1 2 2 2
  spline S193 degree 2 poles (-34.242, 2.3855) (-34.3594, 2.3855) (-34.5714, 2.474) (-34.6516, 2.5543) knots 0 0 0 1 2 2 2
  spline S194 degree 2 poles (-34.6516, 2.5543) (-34.7278, 2.6325) (-34.8204, 2.863) (-34.8204, 2.9907) knots 0 0 0 1 2 2 2
  spline S195 degree 2 poles (-34.8204, 2.9907) (-34.8204, 3.1883) (-34.6537, 3.4682) (-34.4726, 3.5485) knots 0 0 0 1 2 2 2
  spline S196 degree 2 poles (-34.4726, 3.5485) (-34.312, 3.6226) (-33.8756, 3.6781) (-33.6225, 3.6926) knots 0 0 0 1 2 2 2
  line L234 (-33.6225, 3.6926) -> (-33.6225, 3.7543)
  spline S197 degree 2 poles (-33.6225, 3.7543) (-33.6225, 3.8655) (-33.6904, 4.0034) (-33.7521, 4.0425) knots 0 0 0 1 2 2 2
  spline S198 degree 2 poles (-33.7521, 4.0425) (-33.8139, 4.0816) (-33.9909, 4.1063) (-34.0856, 4.1063) knots 0 0 0 1 2 2 2
  spline S199 degree 2 poles (-34.0856, 4.1063) (-34.1967, 4.1063) (-34.4973, 4.0404) (-34.6475, 3.9766) knots 0 0 0 1 2 2 2
  line L235 (-34.6475, 3.9766) -> (-34.666, 3.9766)
  line L236 (-34.666, 3.9766) -> (-34.666, 4.3039)
  spline S200 degree 2 poles (-34.666, 4.3039) (-34.5775, 4.3286) (-34.2461, 4.3903) (-34.0835, 4.3903) knots 0 0 0 1 2 2 2
  spline S201 degree 2 poles (-34.0835, 4.3903) (-33.8859, 4.3903) (-33.6163, 4.3286) (-33.5093, 4.2483) knots 0 0 0 1 2 2 2
  spline S202 degree 2 poles (-33.5093, 4.2483) (-33.4043, 4.1701) (-33.3014, 3.921) (-33.3014, 3.742) knots 0 0 0 1 2 2 2
  line L237 (-33.3014, 3.742) -> (-33.3014, 2.439)
  line L238 (-33.3014, 2.439) -> (-33.6225, 2.439)
  line L239 (-33.6225, 2.439) -> (-33.6225, 2.6407)
  line L240 (-33.6225, 2.9083) -> (-33.6225, 3.4373)
  spline S203 degree 2 poles (-33.6225, 3.4373) (-33.7377, 3.427) (-34.0856, 3.392) (-34.1947, 3.3591) knots 0 0 0 1 2 2 2
  spline S204 degree 2 poles (-34.1947, 3.3591) (-34.3223, 3.32) (-34.489, 3.1574) (-34.489, 3.0133) knots 0 0 0 1 2 2 2
  spline S205 degree 2 poles (-34.489, 3.0133) (-34.489, 2.8486) (-34.3038, 2.6819) (-34.1268, 2.6819) knots 0 0 0 1 2 2 2
  spline S206 degree 2 poles (-34.1268, 2.6819) (-33.9765, 2.6819) (-33.7295, 2.8116) (-33.6225, 2.9083) knots 0 0 0 1 2 2 2
  line L241 (-31.3542, 2.439) -> (-31.6753, 2.439)
  line L242 (-31.6753, 2.439) -> (-31.6753, 3.5258)
  spline S207 degree 2 poles (-31.6753, 3.5258) (-31.6753, 3.6576) (-31.7, 3.884) (-31.737, 3.9519) knots 0 0 0 1 2 2 2
  spline S208 degree 2 poles (-31.737, 3.9519) (-31.7761, 4.0239) (-31.9161, 4.0939) (-32.0355, 4.0939) knots 0 0 0 1 2 2 2
  spline S209 degree 2 poles (-32.0355, 4.0939) (-32.1549, 4.0939) (-32.408, 3.9663) (-32.5295, 3.8634) knots 0 0 0 1 2 2 2
  line L243 (-32.5295, 3.8634) -> (-32.5295, 2.439)
  line L244 (-32.5295, 2.439) -> (-32.8506, 2.439)
  line L245 (-32.8506, 2.439) -> (-32.8506, 4.3451)
  line L246 (-32.8506, 4.3451) -> (-32.5295, 4.3451)
  line L247 (-32.5295, 4.3451) -> (-32.5295, 4.133)
  spline S210 degree 2 poles (-32.5295, 4.133) (-32.3854, 4.2627) (-32.1075, 4.3986) (-31.9511, 4.3986) knots 0 0 0 1 2 2 2
  spline S211 degree 2 poles (-31.9511, 4.3986) (-31.6712, 4.3986) (-31.3542, 4.0281) (-31.3542, 3.6761) knots 0 0 0 1 2 2 2
  line L248 (-31.3542, 3.6761) -> (-31.3542, 2.439)
  spline S212 degree 2 poles (-30.327, 2.402) (-30.5885, 2.402) (-30.8828, 2.7004) (-30.8828, 3.0236) knots 0 0 0 1 2 2 2
  line L249 (-30.8828, 3.0236) -> (-30.8828, 4.0795)
  line L250 (-30.8828, 4.0795) -> (-31.0989, 4.0795)
  line L251 (-31.0989, 4.0795) -> (-31.0989, 4.3451)
  line L252 (-31.0989, 4.3451) -> (-30.8828, 4.3451)
  line L253 (-30.8828, 4.3451) -> (-30.8828, 4.8926)
  line L254 (-30.8828, 4.8926) -> (-30.5617, 4.8926)
  line L255 (-30.5617, 4.8926) -> (-30.5617, 4.3451)
  line L256 (-30.5617, 4.3451) -> (-29.971, 4.3451)
  line L257 (-29.971, 4.3451) -> (-29.971, 4.0795)
  line L258 (-29.971, 4.0795) -> (-30.5617, 4.0795)
  line L259 (-30.5617, 4.0795) -> (-30.5617, 3.1718)
  spline S213 degree 2 poles (-30.5617, 3.1718) (-30.5617, 3.0277) (-30.5514, 2.8692) (-30.5164, 2.8013) knots 0 0 0 1 2 2 2
  spline S214 degree 2 poles (-30.5164, 2.8013) (-30.4876, 2.7416) (-30.3579, 2.6819) (-30.2468, 2.6819) knots 0 0 0 1 2 2 2
  spline S215 degree 2 poles (-30.2468, 2.6819) (-30.1686, 2.6819) (-30.0224, 2.7292) (-29.9895, 2.7437) knots 0 0 0 1 2 2 2
  line L260 (-29.9895, 2.7437) -> (-29.971, 2.7437)
  line L261 (-29.971, 2.7437) -> (-29.971, 2.4555)
  spline S216 degree 2 poles (-29.971, 2.4555) (-30.0615, 2.4308) (-30.2468, 2.402) (-30.327, 2.402) knots 0 0 0 1 2 2 2
  line L262 (-29.407, 2.439) -> (-29.7281, 2.439)
  line L263 (-29.7281, 2.439) -> (-29.7281, 4.3451)
  line L264 (-29.7281, 4.3451) -> (-29.407, 4.3451)
  line L265 (-29.407, 4.3451) -> (-29.407, 2.439)
  line L266 (-29.3843, 4.662) -> (-29.7487, 4.662)
  line L267 (-29.7487, 4.662) -> (-29.7487, 4.9955)
  line L268 (-29.7487, 4.9955) -> (-29.3843, 4.9955)
  line L269 (-29.3843, 4.9955) -> (-29.3843, 4.662)
  spline S217 degree 2 poles (-28.421, 2.3937) (-28.6124, 2.3937) (-28.9438, 2.4967) (-29.0529, 2.5543) knots 0 0 0 1 2 2 2
  line L270 (-29.0529, 2.5543) -> (-29.0529, 2.9145)
  line L271 (-29.0529, 2.9145) -> (-29.0365, 2.9145)
  spline S218 degree 2 poles (-29.0365, 2.9145) (-28.9953, 2.8816) (-28.8841, 2.8034) (-28.7915, 2.7601) knots 0 0 0 1 2 2 2
  spline S219 degree 2 poles (-28.7915, 2.7601) (-28.7112, 2.721) (-28.5136, 2.6634) (-28.4087, 2.6634) knots 0 0 0 1 2 2 2
  spline S220 degree 2 poles (-28.4087, 2.6634) (-28.3325, 2.6634) (-28.1576, 2.6984) (-28.1164, 2.7272) knots 0 0 0 1 2 2 2
  spline S221 degree 2 poles (-28.1164, 2.7272) (-28.0567, 2.7663) (-28.0032, 2.8548) (-28.0032, 2.9454) knots 0 0 0 1 2 2 2
  spline S222 degree 2 poles (-28.0032, 2.9454) (-28.0032, 3.0586) (-28.1267, 3.1759) (-28.2852, 3.215) knots 0 0 0 1 2 2 2
  spline S223 degree 2 poles (-28.2852, 3.215) (-28.3469, 3.2294) (-28.5445, 3.2706) (-28.6289, 3.2932) knots 0 0 0 1 2 2 2
  spline S224 degree 2 poles (-28.6289, 3.2932) (-28.8471, 3.357) (-29.0447, 3.6205) (-29.0447, 3.8078) knots 0 0 0 1 2 2 2
  spline S225 degree 2 poles (-29.0447, 3.8078) (-29.0447, 4.0672) (-28.6557, 4.3903) (-28.3346, 4.3903) knots 0 0 0 1 2 2 2
  spline S226 degree 2 poles (-28.3346, 4.3903) (-28.1761, 4.3903) (-27.855, 4.3121) (-27.7459, 4.2524) knots 0 0 0 1 2 2 2
  line L272 (-27.7459, 4.2524) -> (-27.7459, 3.9087)
  line L273 (-27.7459, 3.9087) -> (-27.7623, 3.9087)
  spline S227 degree 2 poles (-27.7623, 3.9087) (-27.8859, 4.0075) (-28.1864, 4.1207) (-28.3407, 4.1207) knots 0 0 0 1 2 2 2
  spline S228 degree 2 poles (-28.3407, 4.1207) (-28.4992, 4.1207) (-28.7174, 3.9869) (-28.7174, 3.8531) knots 0 0 0 1 2 2 2
  spline S229 degree 2 poles (-28.7174, 3.8531) (-28.7174, 3.7317) (-28.5877, 3.6143) (-28.4437, 3.5773) knots 0 0 0 1 2 2 2
  spline S230 degree 2 poles (-28.4437, 3.5773) (-28.3737, 3.5588) (-28.1967, 3.5217) (-28.0999, 3.4991) knots 0 0 0 1 2 2 2
  spline S231 degree 2 poles (-28.0999, 3.4991) (-27.89, 3.4456) (-27.6759, 3.2006) (-27.6759, 2.9886) knots 0 0 0 1 2 2 2
  spline S232 degree 2 poles (-27.6759, 2.9886) (-27.6759, 2.8651) (-27.7726, 2.6469) (-27.8673, 2.5666) knots 0 0 0 1 2 2 2
  spline S233 degree 2 poles (-27.8673, 2.5666) (-27.9682, 2.4822) (-28.2255, 2.3937) (-28.421, 2.3937) knots 0 0 0 1 2 2 2
  line L274 (-27.7809, 5.2981) -> (-28.1699, 4.6517)
  line L275 (-28.1699, 4.6517) -> (-28.5569, 4.6517)
  line L276 (-28.5569, 4.6517) -> (-28.9459, 5.2981)
  line L277 (-28.9459, 5.2981) -> (-28.6742, 5.2981)
  line L278 (-28.6742, 5.2981) -> (-28.3593, 4.8617)
  line L279 (-28.3593, 4.8617) -> (-28.0443, 5.2981)
  line L280 (-28.0443, 5.2981) -> (-27.7809, 5.2981)
  line L281 (-25.7987, 2.439) -> (-26.2206, 2.439)
  line L282 (-26.2206, 2.439) -> (-26.9287, 3.3591)
  line L283 (-26.9287, 3.3591) -> (-27.0563, 3.2356)
  line L284 (-27.0563, 3.2356) -> (-27.0563, 2.439)
  line L285 (-27.0563, 2.439) -> (-27.3774, 2.439)
  line L286 (-27.3774, 2.439) -> (-27.3774, 5.0922)
  line L287 (-27.3774, 5.0922) -> (-27.0563, 5.0922)
  line L288 (-27.0563, 5.0922) -> (-27.0563, 3.5402)
  line L289 (-27.0563, 3.5402) -> (-26.303, 4.3451)
  line L290 (-26.303, 4.3451) -> (-25.9037, 4.3451)
  line L291 (-25.9037, 4.3451) -> (-26.6858, 3.5485)
  line L292 (-26.6858, 3.5485) -> (-25.7987, 2.439)
  spline S234 degree 2 poles (-24.576, 2.6407) (-24.6151, 2.6119) (-24.7469, 2.509) (-24.8086, 2.4781) knots 0 0 0 1 2 2 2
  spline S235 degree 2 poles (-24.8086, 2.4781) (-24.893, 2.4328) (-25.0515, 2.3855) (-25.1956, 2.3855) knots 0 0 0 1 2 2 2
  spline S236 degree 2 poles (-25.1956, 2.3855) (-25.3129, 2.3855) (-25.5249, 2.474) (-25.6052, 2.5543) knots 0 0 0 1 2 2 2
  spline S237 degree 2 poles (-25.6052, 2.5543) (-25.6814, 2.6325) (-25.774, 2.863) (-25.774, 2.9907) knots 0 0 0 1 2 2 2
  spline S238 degree 2 poles (-25.774, 2.9907) (-25.774, 3.1883) (-25.6073, 3.4682) (-25.4261, 3.5485) knots 0 0 0 1 2 2 2
  spline S239 degree 2 poles (-25.4261, 3.5485) (-25.2656, 3.6226) (-24.8292, 3.6781) (-24.576, 3.6926) knots 0 0 0 1 2 2 2
  line L293 (-24.576, 3.6926) -> (-24.576, 3.7543)